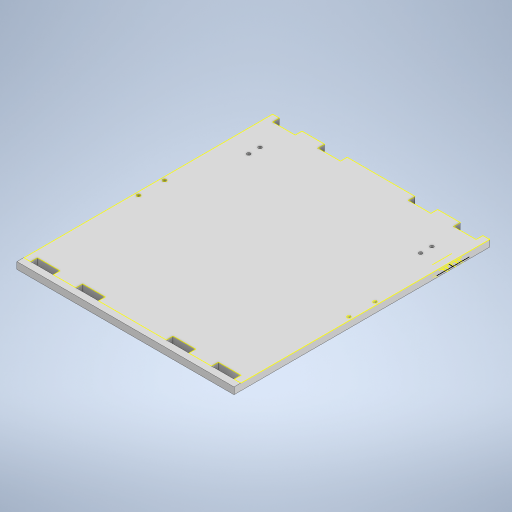
# Autodesk Inventor part: дно_пробитое
Saved by Autodesk Inventor 2024.2 (Build 282272000, 272)
## iProperties
Created: 2025-11-21
Part Number: дно_пробитое
Material: Типовые
Document SubType Name: Modeling
Designer: Zakhar
Density: 1 g/cm^3
Appearance: По умолчанию
Mass: 247.51 g
Surface Area: 882.496 cm^2
Volume: 247.51 cm^3
Author: Zakhar
Autodesk Inventor part; units mm, degrees
ref_plane "YZ Plane" through (0, 0, 0) normal (1, 0, 0) x (0, 1, 0)
ref_plane "XZ Plane" through (0, 0, 0) normal (0, 1, 0) x (-1, 0, 0)
ref_plane "XY Plane" through (0, 0, 0) normal (0, 0, 1) x (1, 0, 0)
sketch "Эскиз1" plane through (0, 0, 0) normal (0, 1, 0) x (-1, 0, 0)
  line L0 (0, 220) -> (192, 220)
  line L1 (192, 220) -> (192, 0)
  line L2 (192, 0) -> (0, 0)
  line L3 (0, 0) -> (0, 220)
  circle A0 centre (11, 217) radius 1.5
  circle A1 centre (181, 217) radius 1.5
  circle A2 centre (5, 3) radius 1.5
  circle A3 centre (187, 3) radius 1.5
  line L4 (186, 6) -> (6, 6)
  line L5 (6, 6) -> (6, 244)
  line L6 (6, 244) -> (186, 244)
  line L7 (186, 244) -> (186, 6)
  dimension "d0" = 192
  dimension "d1" = 170
  dimension "d2" = 220
  dimension "d3" = 11
  dimension "d4" = 3
  dimension "d5" = 3
  dimension "d6" = 3
  dimension "d7" = 3
  dimension "d8" = 3
  dimension "d9" = 5
  dimension "d10" = 3
  dimension "d11" = 3
  dimension "d12" = 5
  dimension "d13" = 3
  dimension "d16" = 238
  dimension "d18" = 180
  dimension "d19" = 6
  dimension "d20" = 6
  constraints: 16 end point, 4 centre point, 4 parallel, 2 horizontal, 2 perpendicular, 1 coincident
  measures "d0" distance of L0.start L0.end
  measures "d1" distance of A0.centre A1.centre
  measures "d2" distance of L2.end L0.start
  measures "d3" distance from line of L3 A0.centre
  measures "d4" diameter of A0
  measures "d5" distance from line of L0 A0.centre
  measures "d6" distance from line of L0 A1.centre
  measures "d7" diameter of A1
  measures "d8" diameter of A2
  measures "d9" distance from line of A2.centre L3
  measures "d10" distance from line of L2 A2.centre
  measures "d11" diameter of A3
  measures "d12" distance from line of L1 A3.centre
  measures "d13" distance from line of L2 A3.centre
  measures "d16" distance of L4.end L5.end
  measures "d18" distance of L4.start L4.end
  measures "d19" distance between parallel lines of L2 L4
  measures "d20" distance between parallel lines of L3 L5
extrude "Выдавливание2" add sketch "Эскиз1" along normal blind 6 contours L0 L5 L4 L7 L1 L2 L3 | L0 L7 L4 L5 | A0 | A1 | A2 | A3
sketch "Эскиз2" plane through (0, 0, 0) normal (0, -1, 0) x (1, 0, 0)
  line L0 (-192, 220) -> (0, 220) projected
  line L1 (-6, 220) -> (-26, 220)
  line L2 (-26, 220) -> (-26, 214)
  line L3 (-26, 214) -> (-6, 214)
  line L4 (-6, 214) -> (-6, 220)
  line L5 (-46, 220) -> (-66, 220)
  line L6 (-66, 220) -> (-66, 214)
  line L7 (-66, 214) -> (-46, 214)
  line L8 (-46, 214) -> (-46, 220)
  line L9 (-186, 220) -> (-166, 220)
  line L10 (-166, 220) -> (-166, 214)
  line L11 (-166, 214) -> (-186, 214)
  line L12 (-186, 214) -> (-186, 220)
  line L13 (-146, 220) -> (-126, 220)
  line L14 (-126, 220) -> (-126, 214)
  line L15 (-126, 214) -> (-146, 214)
  line L16 (-146, 214) -> (-146, 220)
  line L17 (0, 220) -> (0, 0) projected
  line L18 (-192, 0) -> (-192, 220) projected
  point P0 (-66, 217)
  point P1 (-46, 217)
  point P2 (-26, 217)
  point P3 (-146, 217)
  point P4 (-126, 217)
  point P5 (-166, 217)
  point P6 (-186, 217)
  point P7 (-166, 220)
  point P8 (-126, 220)
  dimension "d23" = 6
  dimension "d24" = 20
  dimension "d25" = 6
  dimension "d26" = 20
  dimension "d27" = 20
  dimension "d28" = 20
  dimension "d29" = 20
  dimension "d30" = 20
  dimension "d31" = 6
  constraints: 32 end point, 8 parallel, 7 midpoint, 7 point on line, 4 horizontal, 4 perpendicular
  measures "d23" distance between parallel lines of L4 L17
  measures "d24" distance of L2.end L3.end
  measures "d25" distance between parallel lines of L1 L3
  measures "d26" distance from line of point (-66, 217) L8
  measures "d27" distance of point (-46, 217) point (-26, 217)
  measures "d28" distance of point (-146, 217) point (-126, 217)
  measures "d29" distance of point (-166, 217) point (-146, 217)
  measures "d30" distance of point (-186, 217) point (-166, 217)
  measures "d31" distance from line of L18 point (-186, 217)
extrude "Выдавливание3" cut sketch "Эскиз2" against normal through all
ref_plane "РабПлоскость1" through (-126, 0, 110) normal (0, 0, 1) x (1, 0, 0)
mirror "Зеркальное отражение1" about plane through (-126, 0, 110) normal (0, 0, 1) of "Выдавливание3"
sketch "Эскиз3" plane through (0, 0, 0) normal (0, -1, 0) x (1, 0, 0)
  circle A0 centre (-3, 98.5) radius 1.5
  circle A1 centre (-3, 121.5) radius 1.5
  circle A2 centre (-189, 98.5) radius 1.5
  circle A3 centre (-189, 121.5) radius 1.5
  line L0 (-192, 0) -> (-192, 220) projected
  line L1 (-231.3831, 110) -> (44.2986, 110) projected
  line L2 (0, 220) -> (0, 0) projected
  dimension "d34" = 3
  dimension "d35" = 3
  dimension "d36" = 3
  dimension "d37" = 11.5
  dimension "d38" = 3
  dimension "d39" = 11.5
  dimension "d40" = 3
  dimension "d41" = 3
  dimension "d43" = 11.5
  dimension "d44" = 3
  dimension "d45" = 3
  dimension "d46" = 11.5
  constraints: 4 centre point
  measures "d34" diameter of A3
  measures "d35" diameter of A2
  measures "d36" distance from line of L0 A3.centre
  measures "d37" distance from line of L1 A3.centre
  measures "d38" distance from line of L0 A2.centre
  measures "d39" distance from line of L1 A2.centre
  measures "d40" distance from line of L2 A1.centre
  measures "d41" diameter of A1
  measures "d43" distance from line of L1 A1.centre
  measures "d44" diameter of A0
  measures "d45" distance from line of L2 A0.centre
  measures "d46" distance from line of L1 A0.centre
extrude "Выдавливание4" cut sketch "Эскиз3" against normal blind 10
sketch "Эскиз4" plane through (0, 6, 0) normal (0, 1, 0) x (1, 0, 0)
  line L0 (4.3155, -27.8106) -> (4.3155, -29.0145) projected
  line L1 (4.3155, -43.2101) -> (4.3155, -29.2101) projected
  line L2 (4.3155, -31.8771) -> (4.3155, -40.1101) projected
  line L3 (4.3155, -27.8106) -> (4.3155, -29.0145) projected
  circle A0 centre (-3, -121.5) radius 1.5 projected
  circle A1 centre (-189, -121.5) radius 1.5 projected
  circle A2 centre (-3, -98.5) radius 1.5 projected
  circle A3 centre (-189, -98.5) radius 1.5 projected
  line L4 (-126, 0) -> (-126, -6) projected
  line L5 (-126, -6) -> (-146, -6) projected
  line L6 (-146, -6) -> (-146, 0) projected
  line L7 (-146, 0) -> (-166, 0) projected
  line L8 (-166, 0) -> (-166, -6) projected
  line L9 (-166, -6) -> (-186, -6) projected
  line L10 (-186, -6) -> (-186, 0) projected
  line L11 (-186, 0) -> (-192, 0) projected
  line L12 (-192, 0) -> (-192, -220) projected
  line L13 (-192, -220) -> (-186, -220) projected
  line L14 (-186, -220) -> (-186, -214) projected
  line L15 (-186, -214) -> (-166, -214) projected
  line L16 (-166, -214) -> (-166, -220) projected
  line L17 (-166, -220) -> (-146, -220) projected
  line L18 (-146, -220) -> (-146, -214) projected
  line L19 (-146, -214) -> (-126, -214) projected
  line L20 (-126, -214) -> (-126, -220) projected
  line L21 (-126, -220) -> (-66, -220) projected
  line L22 (-66, -220) -> (-66, -214) projected
  line L23 (-66, -214) -> (-46, -214) projected
  line L24 (-46, -214) -> (-46, -220) projected
  line L25 (-46, -220) -> (-26, -220) projected
  line L26 (-26, -220) -> (-26, -214) projected
  line L27 (-26, -214) -> (-6, -214) projected
  line L28 (-6, -214) -> (-6, -220) projected
  line L29 (-6, -220) -> (0, -220) projected
  line L30 (0, -220) -> (0, 0) projected
  line L31 (0, 0) -> (-6, 0) projected
  line L32 (-6, 0) -> (-6, -6) projected
  line L33 (-6, -6) -> (-26, -6) projected
  line L34 (-26, -6) -> (-26, 0) projected
  line L35 (-26, 0) -> (-46, 0) projected
  line L36 (-46, 0) -> (-46, -6) projected
  line L37 (-46, -6) -> (-66, -6) projected
  line L38 (-66, -6) -> (-66, 0) projected
  line L39 (-66, 0) -> (-126, 0) projected
  line L40 (0, -27.5) -> (0, -30.5) projected
  line L41 (-6, -30.5) -> (-6, -27.5) projected
  line L42 (0, -27.5) -> (0, -30.5) projected
  line L43 (-6, -30.5) -> (-6, -27.5) projected
  line L44 (0, -41.5) -> (0, -44.5) projected
  line L45 (-6, -44.5) -> (-6, -41.5) projected
  line L46 (0, -29) -> (0, -43) projected
  line L47 (-6, -43) -> (-6, -29) projected
  line L48 (0, -41.5) -> (0, -44.5) projected
  line L49 (-6, -44.5) -> (-6, -41.5) projected
  line L50 (4.3155, -22.5218) -> (4.3155, -51.048)
  line L51 (4.9155, -36.9084) -> (0.7155, -36.9084)
  line L52 (4.3155, -22.5218) -> (4.3155, -51.048)
  line L53 (1.3155, -44.914) -> (1.3155, -41.914) projected
  line L54 (4.3155, -44.914) -> (4.3155, -41.914) projected
  line L55 (4.3155, -43.6493) -> (1.3155, -43.6493) projected
  line L56 (4.3155, -40.543) -> (1.3155, -40.543) projected
  line L57 (1.3155, -40.543) -> (1.3155, -46.3135) projected
  line L58 (4.3155, -40.543) -> (4.3155, -46.3135) projected
  line L59 (1.3155, -32.3101) -> (1.3155, -40.543) projected
  line L60 (4.3155, -43.4057) -> (4.3155, -44.6096) projected
  line L61 (4.3155, -32.3101) -> (1.3155, -32.3101) projected
  line L62 (4.3155, -32.3101) -> (4.3155, -40.543) projected
  line L63 (1.3155, -30.9201) -> (1.3155, -27.9201) projected
  line L64 (4.3155, -30.9201) -> (4.3155, -27.9201) projected
  line L65 (1.3155, -26.5206) -> (1.3155, -32.3101) projected
  line L66 (4.3155, -26.5206) -> (4.3155, -32.3101) projected
  line L67 (4.3155, -31.8771) -> (1.3155, -31.8771) projected
  line L68 (4.3155, -28.7709) -> (1.3155, -28.7709) projected
  line L69 (1.3155, -31.8771) -> (1.3155, -40.1101) projected
  line L70 (4.3155, -31.8771) -> (4.3155, -40.1101) projected
  line L71 (1.3155, -43.2101) -> (1.3155, -29.2101) projected
  line L72 (4.3155, -43.2101) -> (4.3155, -29.2101) projected
  line L73 (1.3155, -26.1066) -> (1.3155, -31.8771) projected
  line L74 (4.3155, -26.1066) -> (4.3155, -31.8771) projected
  line L75 (1.3155, -43.4057) -> (1.3155, -44.6096) projected
  line L76 (1.3155, -44.5) -> (1.3155, -41.5) projected
  line L77 (4.3155, -44.5) -> (4.3155, -41.5) projected
  line L78 (4.3155, -43.4057) -> (1.3155, -43.4057) projected
  line L79 (4.3155, -40.1101) -> (1.3155, -40.1101) projected
  line L80 (1.3155, -40.1101) -> (1.3155, -45.8995) projected
  line L81 (4.3155, -40.1101) -> (4.3155, -45.8995) projected
  line L82 (1.3155, -30.5061) -> (1.3155, -27.5061) projected
  line L83 (4.3155, -29.0145) -> (1.3155, -29.0145) projected
  line L84 (4.3155, -27.8106) -> (4.3155, -29.0145) projected
  line L85 (4.3155, -30.5061) -> (4.3155, -27.5061) projected
  line L86 (1.3155, -27.8106) -> (1.3155, -29.0145) projected
  line L87 (4.3155, -41.914) -> (4.3155, -44.914) projected
  line L88 (4.3155, -40.5145) -> (4.3155, -46.3135) projected
  line L89 (4.3155, -43.3697) -> (4.3155, -43.0444) projected
  line L90 (4.3155, -41.5) -> (4.3155, -44.5) projected
  line L91 (4.3155, -40.1005) -> (4.3155, -45.8995) projected
  line L92 (4.3155, -22.2315) -> (4.3155, -52.6365) construction
  line L93 (4.3155, -23.5797) -> (4.3155, -51.7445) construction
  line L94 (4.3155, -35.5823) -> (4.3155, -36.4187) projected
  line L95 (4.3155, -30.9195) -> (4.3155, -41.9147) projected
  line L96 (4.3155, -42.8814) -> (4.3155, -43.61) construction
  line L97 (4.3155, -29.0505) -> (4.3155, -29.2131) projected
  line L98 (4.3155, -29.2101) -> (4.3155, -43.2101) projected
  line L99 (4.3155, -27.8106) -> (4.3155, -44.6096) projected
  line L100 (4.3155, -28.8799) -> (4.3155, -29.6854) construction
  line L101 (4.3155, -29.3758) -> (4.3155, -29.2131) projected
  line L102 (4.3155, -27.9201) -> (4.3155, -30.9201) projected
  line L103 (4.3155, -26.5206) -> (4.3155, -32.3196) projected
  line L104 (4.3155, -27.5061) -> (4.3155, -30.5061) projected
  line L105 (4.3155, -26.1066) -> (4.3155, -31.9056) projected
  line L106 (4.3155, -30.5055) -> (4.3155, -36.0031) projected
  line L107 (4.3155, -41.5007) -> (4.3155, -36.0031) projected
  line L108 (4.3155, -29.6845) -> (4.3155, -30.2653) construction
  point P0 (4.3155, -43.414)
  point P1 (4.3155, -43)
  point P2 (4.3155, -36.2101)
  point P3 (4.3155, -29.4201)
  point P4 (4.3155, -29.0061)
  point P5 (4.3155, -35.9427)
  point P6 (4.3155, -31.8212)
  constraints: 2 end point, 1 horizontal, 31 other
sketch "Эскиз5" plane through (0, 6, 0) normal (0, 1, 0) x (1, 0, 0)
  circle A0 centre (-172, -41) radius 1.5
  circle A1 centre (-172, -31) radius 1.5
  line L0 (-186, -214) -> (-166, -214) projected
  line L1 (-192, 0) -> (-192, -220) projected
  line L2 (-166, -6) -> (-186, -6) projected
  point P0 (0, 0)
  dimension "d49" = 3
  dimension "d52" = 20
  dimension "d53" = 10
  dimension "d54" = 3
  dimension "d57" = 25
  dimension "d58" = 20
  constraints: 2 centre point
  measures "d49" diameter of A0
  measures "d52" distance from line of L1 A1.centre
  measures "d53" distance of A0.centre A1.centre
  measures "d54" diameter of A1
  measures "d57" distance from line of L2 A1.centre
  measures "d58" distance from line of L1 A0.centre
extrude "Выдавливание5" cut sketch "Эскиз5" against normal blind 10
ref_plane "РабПлоскость2" through (-96, 0, 220) normal (1, 0, 0) x (0, 0, -1)
mirror "Зеркальное отражение2" about plane through (-96, 0, 220) normal (1, 0, 0) of "Выдавливание5"
sketch "Эскиз6" plane through (-126, 0, 220) normal (0, 0, 1) x (1, 0, 0)
  line L0 (-66, 6) -> (126, 6)
  line L1 (126, 6) -> (126, 0)
  line L2 (126, 0) -> (-66, 0)
  line L3 (-66, 0) -> (-66, 6)
  line L4 (-66, 6) -> (-60, 6) projected
  line L5 (-60, 6) -> (-60, 0) projected
  line L6 (-60, 0) -> (-66, 0) projected
  line L7 (-66, 0) -> (-66, 6) projected
  line L8 (-40, 6) -> (-20, 6) projected
  line L9 (-20, 6) -> (-20, 0) projected
  line L10 (-20, 0) -> (-40, 0) projected
  line L11 (-40, 0) -> (-40, 6) projected
  line L12 (0, 6) -> (60, 6) projected
  line L13 (60, 6) -> (60, 0) projected
  line L14 (60, 0) -> (0, 0) projected
  line L15 (0, 0) -> (0, 6) projected
  line L16 (80, 6) -> (100, 6) projected
  line L17 (100, 6) -> (100, 0) projected
  line L18 (100, 0) -> (80, 0) projected
  line L19 (80, 0) -> (80, 6) projected
  line L20 (120, 6) -> (126, 6) projected
  line L21 (126, 6) -> (126, 0) projected
  line L22 (126, 0) -> (120, 0) projected
  line L23 (120, 0) -> (120, 6) projected
  line L24 (-66, 6) -> (-60, 6) projected
  line L25 (-60, 6) -> (-60, 0) projected
  line L26 (-60, 0) -> (-66, 0) projected
  line L27 (-40, 6) -> (-20, 6) projected
  line L28 (-20, 6) -> (-20, 0) projected
  line L29 (-20, 0) -> (-40, 0) projected
  line L30 (-40, 0) -> (-40, 6) projected
  line L31 (0, 6) -> (60, 6) projected
  line L32 (60, 6) -> (60, 0) projected
  line L33 (60, 0) -> (0, 0) projected
  line L34 (0, 0) -> (0, 6) projected
  line L35 (80, 6) -> (100, 6) projected
  line L36 (100, 6) -> (100, 0) projected
  line L37 (100, 0) -> (80, 0) projected
  line L38 (80, 0) -> (80, 6) projected
  line L39 (120, 6) -> (126, 6) projected
  line L40 (126, 6) -> (126, 0) projected
  line L41 (126, 0) -> (120, 0) projected
  line L42 (120, 0) -> (120, 6) projected
  line L43 (-66, 6) -> (-60, 6) projected
  line L44 (-60, 6) -> (-60, 0) projected
  line L45 (-60, 0) -> (-66, 0) projected
  line L46 (-40, 6) -> (-20, 6) projected
  line L47 (-20, 6) -> (-20, 0) projected
  line L48 (-20, 0) -> (-40, 0) projected
  line L49 (-40, 0) -> (-40, 6) projected
  line L50 (0, 6) -> (60, 6) projected
  line L51 (60, 6) -> (60, 0) projected
  line L52 (60, 0) -> (0, 0) projected
  line L53 (0, 0) -> (0, 6) projected
  line L54 (80, 6) -> (100, 6) projected
  line L55 (100, 6) -> (100, 0) projected
  line L56 (100, 0) -> (80, 0) projected
  line L57 (80, 0) -> (80, 6) projected
  line L58 (120, 6) -> (126, 6) projected
  line L59 (126, 6) -> (126, 0) projected
  line L60 (126, 0) -> (120, 0) projected
  line L61 (120, 0) -> (120, 6) projected
  line L62 (120, 6) -> (126, 6) projected
  line L63 (126, 0) -> (126, 6) projected
  line L64 (120, 0) -> (126, 0) projected
  line L65 (-66, 0) -> (-66, 6) projected
  line L66 (-66, 0) -> (-66, 6) projected
  constraints: 6 end point, 3 collinear, 3 horizontal, 1 parallel, 1 perpendicular, 3 other
extrude "Выдавливание6" add sketch "Эскиз6" along normal blind 6
equation "\"d26\" = d24"
equation "\"d27\" = d24"
equation "\"d28\" = d24"
equation "\"d29\" = d24"
equation "\"d30\" = d24"
equation "\"d39\" = d37"
equation "\"d43\" = d37"
equation "\"d46\" = d37"
